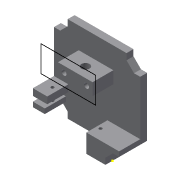
# Autodesk Inventor part: 20_Cube_Insert_RaspiCam_v3
Saved by Autodesk Inventor 2019.4 (Build 234330000, 330)
## iProperties
Created: 2019-07-01
Part Number: 20_Cube_Insert_RaspiCam_v3
Material: Generic
Document SubType Name: Modeling
Designer: diederichbenedict
Density: 1 g/cm^3
Appearance: Default
Author: diederichbenedict
Autodesk Inventor part; units mm, degrees
ref_plane "YZ Plane" through (0, 0, 0) normal (1, 0, 0) x (0, 1, 0)
ref_plane "Work Plane1" through (0, 0, 10) normal (0, 0, 1) x (1, 0, 0)
sketch "Sketch1" plane through (0, 0, 10) normal (0, 0, 1) x (1, 0, 0)
  line L0 (-4.0299, -0.3538) -> (-2.2322, 1.4439) construction
  arc A0 (-1.4439, 2.2322) -> (-2.2322, 1.4439) centre (-0.9299, 0.9299) ccw construction
  line L1 (-1.4439, 2.2322) -> (0.3538, 4.0299) construction
  line L2 (-37.8299, 42.2137) -> (-37.8299, 45.8299) construction
  line L3 (-37.8299, 45.8299) -> (-4.0299, 45.8299) construction
  line L4 (-4.0299, 45.8299) -> (-4.0299, 42.2137) construction
  line L5 (-4.0299, 4.0299) -> (0.3538, 4.0299) projected
  circle A1 centre (-20.9299, 20.9299) radius 17.5 construction
  line L6 (-20.9299, 58.9723) -> (17.1124, 20.9299) construction
  line L7 (17.1124, 20.9299) -> (-20.9299, -17.1124) construction
  line L8 (-20.9299, -17.1124) -> (-58.9723, 20.9299) construction
  line L9 (-58.9723, 20.9299) -> (-20.9299, 58.9723) construction
  line L10 (-20.9299, 58.9723) -> (-20.9299, -17.1124) construction
  line L11 (17.1124, 20.9299) -> (-58.9723, 20.9299) construction
  line L12 (-20.9299, 58.9723) -> (32.8701, 58.9723) construction
  line L13 (-43.2198, 43.4299) -> (1.7802, 43.4299) construction
  line L14 (1.7802, 43.4299) -> (1.7802, -1.5701) construction
  line L15 (1.7802, -1.5701) -> (-43.2198, -1.5701) construction
  line L16 (-43.2198, -1.5701) -> (-43.2198, 43.4299) construction
  line L17 (-43.2198, 5.1774) -> (-43.2198, 36.6824)
  line L18 (-43.2198, 36.6824) -> (-36.4723, 43.4299)
  line L19 (-36.4723, 43.4299) -> (-5.3876, 43.4299)
  line L20 (-5.3876, 43.4299) -> (1.7802, 36.2621)
  line L21 (1.7802, 36.2621) -> (1.7802, 5.5977)
  line L22 (1.7802, 5.5977) -> (-5.3876, -1.5701)
  line L23 (-5.3876, -1.5701) -> (-36.4723, -1.5701)
  line L24 (-36.4723, -1.5701) -> (-43.2198, 5.1774)
  line L25 (-4.0299, 42.2137) -> (-37.8299, 42.2137) projected
  line L26 (-4.0299, -0.3538) -> (-4.0299, 4.0299) projected
  circle A2 centre (-20.7198, 20.9299) radius 7.0417 construction
  arc A3 (-7.3745, 3.5) -> (-34.4854, 3.5) centre (-20.9299, 0) ccw construction
  arc A4 (-11.4668, 9.7661) -> (-30.4087, 10.1422) centre (-20.7198, 20.9299) ccw
  line L27 (-30.5806, 10.1422) -> (-30.4087, 10.1422)
  line L28 (-30.4087, 10.1422) -> (-30.4087, 1.6029)
  line L29 (-30.4087, 1.6029) -> (-11.4668, 1.6029)
  line L30 (-11.4668, 1.6029) -> (-11.4668, 9.7661)
  line L31 (-43.2198, 43.4299) -> (-10.4667, 10.6769) construction
  line L32 (-8.5595, 8.5517) -> (1.7802, -1.5701) construction
  line L33 (1.7802, 43.4299) -> (-25.699, 15.9507) construction
  line L34 (-30.9728, 10.6769) -> (-43.2198, -1.5701) construction
  point P0 (-37.8299, 4.0299)
  dimension "d18" = 53.8
  dimension "d19" = 45
  dimension "d20" = 53.8
  dimension "d21" = 45
  dimension "d22" = 45
  dimension "d68" = 29
  constraints: 54 end point, 20 point on line, 6 parallel, 5 point on circle, 4 perpendicular, 3 horizontal, 2 midpoint, 1 centre point, 1 coincident, 1 equal length, 5 other
  measures "d18" distance of L6.start L6.end
  measures "d19" angle of L6 L12
  measures "d20" distance of L6.end L7.end
  measures "d21" distance of L14.end L15.end
  measures "d22" distance of L13.end L14.end
  measures "d68" diameter of A4
extrude "Extrusion1" add sketch "Sketch1" along normal blind 4 contours L26 L22 L23 L24 L17 L18 L25 L20 L21 L5 | L5 L22 L26 | L25 L18 L19 L20 | L30 L29 L28 A4
sketch "Sketch3" plane through (0, 0, 10) normal (0, 0, -1) x (-1, 0, 0)
  line L0 (37.8299, -0.4701) -> (37.8299, 4.0299) construction
  line L1 (4.0299, 4.0299) -> (4.0299, -0.4701) construction
  line L2 (37.8299, -0.4701) -> (37.8299, 1.1886) construction
  line L3 (4.0299, -3.9701) -> (4.0299, -0.3538) construction
  line L4 (45.8299, 4.0299) -> (42.2137, 4.0299) construction
  line L5 (-0.3538, 4.0299) -> (-3.9701, 4.0299) construction
  line L6 (-3.9701, 37.8299) -> (-0.3538, 37.8299) construction
  line L7 (4.0299, 42.2137) -> (4.0299, 45.8299) construction
  line L8 (37.8299, 45.8299) -> (37.8299, 42.2137) construction
  line L9 (42.2137, 37.8299) -> (45.8299, 37.8299) construction
  line L10 (37.8299, 37.7299) -> (45.8299, 37.7299)
  line L11 (45.8299, 37.7299) -> (45.8299, 4.1299)
  line L12 (45.8299, 4.1299) -> (37.8299, 4.1299)
  line L13 (37.8299, 4.1299) -> (37.8299, 37.7299)
  line L14 (37.7299, 4.0299) -> (4.1299, 4.0299)
  line L15 (4.1299, 4.0299) -> (4.1299, -3.9701)
  line L16 (4.1299, -3.9701) -> (37.7299, -3.9701)
  line L17 (37.7299, -3.9701) -> (37.7299, 4.0299)
  line L18 (4.0299, 4.1299) -> (-3.9701, 4.1299)
  line L19 (-3.9701, 4.1299) -> (-3.9701, 37.7299)
  line L20 (-3.9701, 37.7299) -> (4.0299, 37.7299)
  line L21 (4.0299, 37.7299) -> (4.0299, 4.1299)
  line L22 (4.1299, 37.8299) -> (37.7299, 37.8299)
  line L23 (37.7299, 37.8299) -> (37.7299, 45.8299)
  line L24 (37.7299, 45.8299) -> (4.1299, 45.8299)
  line L25 (4.1299, 45.8299) -> (4.1299, 37.8299)
  point P0 (0, 0)
  dimension "d23" = 0.1
  dimension "d24" = 0.1
  dimension "d25" = 0.1
  dimension "d26" = 0.1
  dimension "d27" = 0.1
  constraints: 32 end point, 8 parallel, 4 horizontal, 4 perpendicular, 3 point on line
  measures "d23" distance between parallel lines of L8 L23
  measures "d24" distance between parallel lines of L7 L25
  measures "d25" distance between parallel lines of L6 L20
  measures "d26" distance between parallel lines of L5 L18
  measures "d27" distance between parallel lines of L1 L15
extrude "Extrusion3" add sketch "Sketch3" against normal up to surface (4 mm away)
sketch "Skizze12" plane through (0, 0, 10) normal (0, 0, -1) x (-1, 0, 0)
  line L0 (-0.3124, 4.1299) -> (4.1299, -0.3124) projected
  line L1 (4.1299, -0.3124) -> (4.1299, -3.9701) projected
  line L2 (4.1299, -3.9701) -> (37.7299, -3.9701) construction
  line L3 (37.7299, -3.9701) -> (37.7299, -0.3124) projected
  line L4 (37.7299, -0.3124) -> (42.1723, 4.1299) projected
  line L5 (45.8299, 4.1299) -> (42.1723, 4.1299) projected
  line L6 (45.8299, 37.7299) -> (45.8299, 4.1299) construction
  line L7 (42.1723, 37.7299) -> (45.8299, 37.7299) projected
  line L8 (42.1723, 37.7299) -> (37.7299, 42.1723) projected
  line L9 (37.7299, 42.1723) -> (37.7299, 45.8299) projected
  line L10 (37.7299, 45.8299) -> (4.1299, 45.8299) construction
  line L11 (4.1299, 45.8299) -> (4.1299, 42.1723) projected
  line L12 (4.1299, 42.1723) -> (-0.3124, 37.7299) projected
  line L13 (-3.9701, 37.7299) -> (-0.3124, 37.7299) projected
  line L14 (-3.9701, 4.1299) -> (-3.9701, 37.7299) construction
  line L15 (-0.3124, 4.1299) -> (-3.9701, 4.1299) projected
  line L16 (37.9299, -4.1701) -> (3.9299, -4.1701) construction
  line L17 (3.9299, -4.1701) -> (3.9299, -0.3953)
  line L18 (3.9299, -0.3953) -> (-0.3953, 3.9299)
  line L19 (-0.3953, 3.9299) -> (-4.1701, 3.9299)
  line L20 (-4.1701, 3.9299) -> (-4.1701, 37.9299) construction
  line L21 (-4.1701, 37.9299) -> (-0.3953, 37.9299)
  line L22 (-0.3953, 37.9299) -> (3.9299, 42.2551)
  line L23 (3.9299, 42.2551) -> (3.9299, 46.0299)
  line L24 (3.9299, 46.0299) -> (37.9299, 46.0299) construction
  line L25 (37.9299, 46.0299) -> (37.9299, 42.2551)
  line L26 (37.9299, 42.2551) -> (42.2551, 37.9299)
  line L27 (42.2551, 37.9299) -> (46.0299, 37.9299)
  line L28 (46.0299, 37.9299) -> (46.0299, 3.9299) construction
  line L29 (46.0299, 3.9299) -> (42.2551, 3.9299)
  line L30 (42.2551, 3.9299) -> (37.9299, -0.3953)
  line L31 (37.9299, -0.3953) -> (37.9299, -4.1701)
  line L32 (-3.9701, 37.7299) -> (-3.9701, 37.9299)
  line L33 (37.7299, 45.8299) -> (4.1299, 45.8299) projected
  line L34 (4.1299, 45.8299) -> (3.9299, 45.8299)
  line L35 (37.7299, 45.8299) -> (37.9299, 45.8299)
  line L36 (45.8299, 37.7299) -> (45.8299, 37.9299)
  line L37 (45.8299, 4.1299) -> (45.8299, 3.9299)
  line L38 (37.7299, -3.9701) -> (37.9299, -3.9701)
  line L39 (4.1299, -3.9701) -> (3.9299, -3.9701)
  line L40 (-3.9701, 4.1299) -> (-3.9701, 3.9299)
  point P0 (0, 0)
  dimension "d65" = 0.2
  constraints: 48 end point, 13 point on line, 2 perpendicular, 1 vertical, 15 other
  measures "d65" distance between parallel lines of L2 L16
extrude "IM_offset" add sketch "Skizze12" against normal up to surface (4 mm away)
sketch "Sketch15" plane through (0, 0, 14) normal (0, 0, 1) x (1, 0, 0)
  line L0 (-16.2999, 13.4299) -> (-16.2999, 9.2299) projected
  line L1 (-16.2999, 13.4299) -> (-19.9879, 13.4299) projected
  line L2 (-21.5499, 13.4299) -> (-19.9879, 13.4299) projected
  line L3 (-23.112, 13.4299) -> (-21.5499, 13.4299) projected
  line L4 (-23.112, 13.4299) -> (-37.0999, 13.4299) projected
  line L5 (-37.0999, 13.4299) -> (-37.0999, 9.2299) projected
  line L6 (-41.8999, 9.2299) -> (-37.0999, 9.2299) projected
  line L7 (-41.8999, 9.2299) -> (-41.8999, 6.7299) projected
  line L8 (-41.8999, 6.7299) -> (-11.4999, 6.7299) projected
  line L9 (-11.4999, 9.2299) -> (-11.4999, 6.7299) projected
  line L10 (-16.2999, 9.2299) -> (-11.4999, 9.2299) projected
  line L11 (3.9701, 37.9299) -> (3.9701, 3.9299) projected
  line L12 (0.3953, 37.9299) -> (3.9701, 37.9299) projected
  line L13 (-3.9299, 42.2551) -> (0.3953, 37.9299) projected
  line L14 (-3.9299, 45.8299) -> (-3.9299, 42.2551) projected
  line L15 (-37.9299, 45.8299) -> (-3.9299, 45.8299) projected
  line L16 (-37.9299, 42.2551) -> (-37.9299, 45.8299) projected
  line L17 (-42.2551, 37.9299) -> (-37.9299, 42.2551) projected
  line L18 (-45.8299, 37.9299) -> (-42.2551, 37.9299) projected
  line L19 (-45.8299, 3.9299) -> (-45.8299, 37.9299) projected
  line L20 (-42.2551, 3.9299) -> (-45.8299, 3.9299) projected
  line L21 (-37.9299, -0.3953) -> (-42.2551, 3.9299) projected
  line L22 (-37.9299, -3.9701) -> (-37.9299, -0.3953) projected
  line L23 (-3.9299, -3.9701) -> (-37.9299, -3.9701) projected
  line L24 (-3.9299, -0.3953) -> (-3.9299, -3.9701) projected
  line L25 (0.3953, 3.9299) -> (-3.9299, -0.3953) projected
  line L26 (3.9701, 3.9299) -> (0.3953, 3.9299) projected
  line L27 (-45.8299, 3.9299) -> (-38.9491, 3.9299)
  line L28 (-38.9491, 3.9299) -> (-38.9491, 6.7299)
  line L29 (-38.9491, 6.7299) -> (-45.8299, 6.7299)
  line L30 (-45.8299, 6.7299) -> (-45.8299, 3.9299)
  line L31 (3.9701, 3.9299) -> (0.3953, 3.9299) projected
  line L32 (-14.947, 6.7299) -> (3.9701, 6.7299)
  line L33 (3.9701, 6.7299) -> (3.9701, 3.9299)
  line L34 (3.9701, 3.9299) -> (-14.947, 3.9299)
  line L35 (-14.947, 3.9299) -> (-14.947, 6.7299)
  line L36 (0.3953, 3.9299) -> (-3.9299, -0.3953)
  line L37 (-3.9299, -0.3953) -> (-3.9299, -3.9701)
  line L38 (-3.9299, -3.9701) -> (-37.9299, -3.9701) projected
  line L39 (-3.9299, -3.9701) -> (-14.947, -3.9701)
  line L40 (-14.947, 3.9299) -> (-14.947, -3.9701)
  line L41 (-45.8299, 3.9299) -> (-45.8299, 37.9299) projected
  line L42 (-45.8299, 9.5618) -> (-37.5128, 9.5618)
  line L43 (-37.5128, 9.5618) -> (-37.5128, 13.4299)
  line L44 (-37.5128, 13.4299) -> (-45.8299, 13.4299)
  line L45 (-45.8299, 13.4299) -> (-45.8299, 9.5618)
  point P0 (0, 0)
  constraints: 32 end point, 6 parallel, 4 perpendicular, 4 point on line, 3 horizontal, 1 vertical
ref_plane "Work Plane4" through (-41.8999, 11.7299, 26.2) normal (0, 0, 1) x (1, 0, 0)
extrude "Extrusion13" add sketch "Sketch15" along normal up to surface (12.2 mm away) contours L32 L11 L26 L34 L35 L8 | L28 L27 L20 L19 L29 L8 | L34 L25 L24 L23 L40 | L19 L44 L43 L42
sketch "Sketch16" plane through (-45.8299, -3.9701, 10) normal (0, -1, 0) x (1, 0, 0)
  circle A0 centre (5.23, 10.1) radius 0.8388 projected
  circle A1 centre (5.23, 10.1) radius 1.5765 projected
  circle A2 centre (33.03, 10.1) radius 2.4 projected
  point P0 (45.8299, -10)
hole "Hole1" at (-40.5999, -3.9701, 20.1) at (-12.7999, -3.9701, 20.1) direction (0, 1, 0) diameter 1.8 end through all
sketch "Sketch17" plane through (0, 0, 14) normal (0, 0, 1) x (1, 0, 0)
  line L0 (-18.1603, 25.8799) -> (-22.3637, 25.8799) projected
  line L1 (-22.3637, 25.8799) -> (-47.0707, 25.8799) projected
  line L2 (-19.1999, 18.8799) -> (-19.1999, 25.8799)
  line L3 (-23.8999, 18.8799) -> (-23.8999, 25.8799)
  line L4 (-11.5499, 26.4651) -> (-31.5499, 26.4651)
  line L5 (-31.5499, 26.4651) -> (-31.5499, 33.4651)
  line L6 (-31.5499, 33.4651) -> (-11.5499, 33.4651)
  line L7 (-11.5499, 33.4651) -> (-11.5499, 26.4651)
  point P0 (0, 0)
  dimension "d82" = 20
  dimension "d83" = 7
  dimension "d84" = 7.65
  constraints: 12 end point, 2 parallel, 2 vertical, 1 horizontal, 1 perpendicular, 4 other
  measures "d82" distance of L5.end L6.end
  measures "d83" distance of L4.end L5.end
  measures "d84" distance between parallel lines of L7 L2
extrude "Extrusion14" add sketch "Sketch17" along normal blind 12
sketch "Sketch18" plane through (-31.5499, 33.4651, 14) normal (0, 1, 0) x (1, 0, 0)
  circle A0 centre (10, -6.1) radius 2.35 projected
  point P0 (31.5499, 14)
extrude "Extrusion15" cut sketch "Sketch18" against normal blind 12
sketch "Sketch19" plane through (0, 0, 26) normal (0, 0, 1) x (1, 0, 0)
  line L0 (-31.5499, 26.4651) -> (-11.5499, 26.4651) projected
  line L1 (-11.5499, 26.4651) -> (-11.5499, 33.4651) projected
  line L2 (-11.5499, 33.4651) -> (-31.5499, 33.4651) projected
  line L3 (-31.5499, 33.4651) -> (-31.5499, 26.4651) projected
  circle A0 centre (-15.0499, 29.9651) radius 1.45
  circle A1 centre (-28.0499, 29.9651) radius 1.45
  point P0 (0, 0)
  dimension "d89" = 2.9
  dimension "d90" = 3.5
  dimension "d91" = 3.5
  dimension "d92" = 2.9
  dimension "d93" = 3.5
  constraints: 2 centre point
  measures "d89" diameter of A0
  measures "d90" distance from line of A0.centre L0
  measures "d91" distance from line of L1 A0.centre
  measures "d92" diameter of A1
  measures "d93" distance from line of A1.centre L3
extrude "Extrusion16" cut sketch "Sketch19" against normal through all contours A0 | A1
sketch "Sketch20" plane through (0, 0, 26) normal (0, 0, 1) x (1, 0, 0)
  line L0 (-9.7781, 37.8674) -> (-41.4214, 37.8674)
  line L1 (-41.4214, 37.8674) -> (-41.4214, 22.8936)
  line L2 (-41.4214, 22.8936) -> (-9.7781, 22.8936)
  line L3 (-9.7781, 22.8936) -> (-9.7781, 37.8674)
  point P0 (0, 0)
  constraints: 8 end point, 2 parallel, 1 horizontal, 1 perpendicular
body "Solid1"
